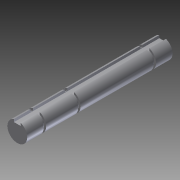
# Autodesk Inventor part: lower box upper shaft
Saved by Autodesk Inventor 2012 (Build 160160000, 160)
## iProperties
Created: 2012-07-06
Part Number: lower box upper shaft
Material: Default
Document SubType Name: Modeling
Designer: Bryce
Density: 1 g/cm^3
Author: Bryce
Autodesk Inventor part; units mm, degrees
sketch "Sketch1" plane through (0, 0, 0) normal (0, 0, 1) x (1, 0, 0)
  circle A0 centre (0, 0) radius 4.7625
  line L0 (-1.5875, 6.35) -> (1.5875, 6.35)
  line L1 (1.5875, 6.35) -> (1.5875, 3.175)
  line L2 (1.5875, 3.175) -> (-1.5875, 3.175)
  line L3 (-1.5875, 3.175) -> (-1.5875, 6.35)
  dimension "d0" = 9.525
  dimension "d16" = 3.175
  dimension "d17" = 3.175
  dimension "d18" = 1.5875
  dimension "d19" = 6.35
  constraints: 8 end point, 2 parallel, 1 centre point, 1 coincident, 1 horizontal, 1 perpendicular
  measures "d0" diameter of A0
  measures "d16" distance of L0.start L0.end
  measures "d17" distance of L0.end L1.end
  measures "d18" distance from line of point (0, 0) L1
  measures "d19" distance from line of point (0, 0) L0
extrude "Extrusion1" add sketch "Sketch1" along normal blind 69.85 contours A0 L3 L2 L1 | L1 L2 L3 A0
ref_plane "Work Plane1" through (0, 0, 61.9125) normal (0, 0, 1) x (1, 0, 0)
sketch "Sketch2" plane through (0, 0, 61.9125) normal (0, 0, 1) x (1, 0, 0)
  circle A0 centre (0, 0) radius 3.81
  circle A1 centre (0, 0) radius 4.7625 projected
  dimension "d4" = 7.62
  constraints: 1 centre point, 1 coincident
  measures "d4" diameter of A0
extrude "Extrusion2" cut sketch "Sketch2" against normal blind 1.143
ref_plane "Work Plane2" through (0, 0, 7.9375) normal (0, 0, -1) x (-1, 0, 0)
sketch "Sketch3" plane through (0, 0, 7.9375) normal (0, 0, -1) x (-1, 0, 0)
  circle A0 centre (0, 0) radius 3.81 projected
  circle A1 centre (0, 0) radius 4.7625 projected
extrude "Extrusion3" cut sketch "Sketch3" against normal blind 1.143
ref_plane "Work Plane3" through (0, 0, 44.2214) normal (0, 0, 1) x (1, 0, 0)
sketch "Sketch4" plane through (0, 0, 44.2214) normal (0, 0, 1) x (1, 0, 0)
  circle A0 centre (0, 0) radius 3.81 projected
  circle A1 centre (0, 0) radius 4.7625 projected
extrude "Extrusion4" cut sketch "Sketch4" along normal blind 1.143
ref_plane "Work Plane4" through (0, 0, 68.1736) normal (0, 0, 1) x (1, 0, 0)
extrude "Extrusion6" cut sketch "Sketch1" along normal through all contours L1 L2 L3 A0 | A0 L3 L0 L1 picked at (-0.1794, 3.694)
equation "\"d17\" = d16"
equation "\"d18\" = 0.5 * d16"
body "Solid1"
